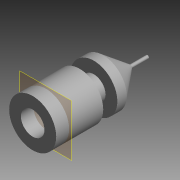
# Autodesk Inventor part: Nozzle
Saved by Autodesk Inventor 2015 (Build 190159000, 159)
## iProperties
Created: 2015-01-06
Part Number: Nozzle
Material: Generic
Document SubType Name: Modeling
Designer: ice
Density: 1 g/cm^3
Appearance: Default
Mass: 1.02114 g
Surface Area: 9.24729 cm^2
Volume: 1.02114 cm^3
Author: ice
Autodesk Inventor part; units mm, degrees
ref_plane "YZ Plane" through (0, 0, 0) normal (1, 0, 0) x (0, 1, 0)
ref_plane "XZ Plane" through (0, 0, 0) normal (0, 1, 0) x (-1, 0, 0)
ref_plane "XY Plane" through (0, 0, 0) normal (0, 0, 1) x (1, 0, 0)
sketch "Sketch1" plane through (0, 0, 0) normal (0, 0, 1) x (1, 0, 0)
  line L0 (-2.5, -0.8) -> (-2.5, -6)
  line L1 (-2.5, -6) -> (-5, -6)
  line L2 (-5, -6) -> (-5, 4)
  line L3 (-5, 4) -> (-2.5, 4)
  line L4 (-2.5, 4) -> (-2.5, 7)
  line L5 (-2.5, 7) -> (-5, 7)
  line L6 (-5, 7) -> (-5, 9)
  line L7 (-0.35, 14.8125) -> (-5, 9)
  line L8 (0, 14.375) -> (0, 0)
  line L9 (0, 14.375) -> (0, 18.375)
  line L10 (-0.15, 18.375) -> (-0.35, 18.375)
  line L11 (-0.35, 18.375) -> (-0.35, 14.8125)
  line L12 (-1, 0) -> (-1, 12.1943)
  line L13 (-0.15, 18.375) -> (-0.15, 13.0443)
  arc A0 (-0.15, 13.0443) -> (-1, 12.1943) centre (-0.15, 12.1943) ccw
  line L14 (-2.5, -0.8) -> (-1, -0.8)
  line L15 (-1, -0.8) -> (-1, 0)
  point P0 (-1, 14)
  point P1 (-0.7, 14.375)
  dimension "d2" = 2.5
  dimension "d3" = 10
  dimension "d4" = 2.5
  dimension "d5" = 3
  dimension "d7" = 2
  dimension "d54" = 24.375
  dimension "d55" = 3.5625
  dimension "d56" = 2.5
  dimension "d57" = 1
  dimension "d58" = 5.8125
  dimension "d59" = 0.35
  dimension "d60" = 0.15
  dimension "d61" = 5.2
  dimension "d62" = 13.8443
  constraints: 32 end point, 7 point on line, 4 perpendicular, 2 point on circle, 1 centre point, 1 vertical
  measures "d2" distance of L0.end L1.end
  measures "d3" distance of L1.end L2.end
  measures "d4" distance of L2.end L3.end
  measures "d5" distance of L3.end L4.end
  measures "d7" distance of L5.end L6.end
  measures "d54" vertical distance of L0.end L10.start
  measures "d55" distance of L7.start L10.end
  measures "d56" horizontal distance of L8.end L0.end
  measures "d57" horizontal distance of L8.end L14.end
  measures "d58" vertical distance of L6.end L7.start
  measures "d59" distance of L9.end L10.end
  measures "d60" distance of L10.start L9.end
  measures "d61" distance of L0.end L0.start
  measures "d62" vertical distance of L14.end L13.end
revolve "Revolution1" add sketch "Sketch1" angle 360 about axis through (0, 14.375, 0) along (0, -1, 0)
ref_plane "Work Plane1" through (0, -3.25, 0) normal (0, -1, 0) x (1, 0, 0)
sketch "Sketch2" plane through (0, -3.25, 0) normal (0, -1, 0) x (1, 0, 0)
  point P0 (0, 0)
body "Solid1"
